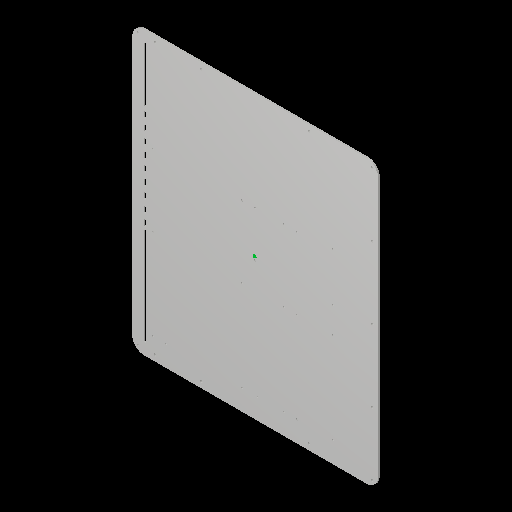
# Autodesk Inventor part: right_panel
Saved by Autodesk Inventor 2022 (Build 260153000, 153)
## iProperties
Created: 2019-10-14
Part Number: right_panel
Material: アルミニウム 6061
Document SubType Name: Modeling
Designer: gisen
Density: 2.7 g/cm^3
Appearance: アルミニウム - フラット
Author: gisen
Autodesk Inventor part; units mm, degrees
ref_plane "YZ Plane" through (0, 0, 0) normal (1, 0, 0) x (0, 1, 0)
ref_plane "XZ Plane" through (0, 0, 0) normal (0, 1, 0) x (-1, 0, 0)
ref_plane "XY Plane" through (0, 0, 0) normal (0, 0, 1) x (1, 0, 0)
sketch "スケッチ1" plane through (0, 0, 0) normal (0, 0, 1) x (1, 0, 0)
  line L0 (-193.5, -245) -> (193.5, -245)
  line L1 (213.5, -225) -> (213.5, 225)
  line L2 (193.5, 245) -> (-193.5, 245)
  line L3 (-213.5, 225) -> (-213.5, -225)
  line L4 (-213.5, -245) -> (213.5, 245) construction
  line L5 (213.5, -245) -> (-213.5, 245) construction
  circle A0 centre (-203.5, 235) radius 2.25
  circle A1 centre (203.5, 235) radius 2.25
  circle A2 centre (-203.5, -235) radius 2.25
  circle A3 centre (203.5, -235) radius 2.25
  arc A4 (-193.5, 245) -> (-213.5, 225) centre (-193.5, 225) ccw
  arc A5 (213.5, 225) -> (193.5, 245) centre (193.5, 225) ccw
  arc A6 (193.5, -245) -> (213.5, -225) centre (193.5, -225) ccw
  arc A7 (-213.5, -225) -> (-193.5, -245) centre (-193.5, -225) ccw
  point P0 (0, 0)
  dimension "d0" = 427
  dimension "d1" = 490
  dimension "d2" = 4.5
  dimension "d3" = 10
  dimension "d4" = 10
  dimension "d5" = 10
  dimension "d6" = 10
  dimension "d7" = 10
  dimension "d8" = 10
  dimension "d9" = 10
  dimension "d10" = 10
  dimension "d11" = 20
  constraints: 12 end point, 8 centre point, 8 point on circle, 8 point on line, 8 tangent, 6 equal radius, 2 midpoint, 2 parallel, 1 horizontal, 1 perpendicular
  measures "d0" distance of L5.end L4.end
  measures "d1" distance of L4.end L5.start
  measures "d2" diameter of A0
  measures "d3" distance from line of A0.centre L2
  measures "d4" distance from line of L3 A0.centre
  measures "d5" distance from line of A1.centre L2
  measures "d6" distance from line of L1 A1.centre
  measures "d7" distance from line of L1 A3.centre
  measures "d8" distance from line of L0 A3.centre
  measures "d9" distance from line of L0 A2.centre
  measures "d10" distance from line of L3 A2.centre
  measures "d11" radius of A4
extrude "押し出し1" add sketch "スケッチ1" along normal blind 3
sketch "スケッチ2" plane through (0, 0, 3) normal (0, 0, 1) x (1, 0, 0)
  circle A0 centre (49.592, 72.9258) radius 1.6
  circle A1 centre (-22.798, 72.9258) radius 1.6
  circle A2 centre (-177.738, 72.9258) radius 1.6
  circle A3 centre (-177.738, -51.5342) radius 1.6
  circle A4 centre (-154.878, -209.0142) radius 1.6
  circle A5 centre (-22.798, -209.0142) radius 1.6
  circle A6 centre (49.592, -209.0142) radius 1.6
  circle A7 centre (49.592, -51.5342) radius 1.6
  circle A8 centre (-22.798, -51.5342) radius 1.6
  circle A9 centre (49.592, -209.0142) radius 2.25 projected
  circle A10 centre (-154.878, -209.0142) radius 2.25 projected
  circle A11 centre (49.592, -51.5342) radius 2.25 projected
  circle A12 centre (49.592, 72.9258) radius 2.25 projected
  circle A13 centre (-22.798, -209.0142) radius 2.25 projected
  circle A14 centre (-22.798, -51.5342) radius 2.25 projected
  circle A15 centre (-22.798, 72.9258) radius 2.25 projected
  circle A16 centre (-177.738, -51.5342) radius 2.25 projected
  circle A17 centre (-177.738, 72.9258) radius 2.25 projected
  point P0 (0, 0)
  dimension "d14" = 3.2
  constraints: 9 centre point, 9 concentric, 8 equal radius
  measures "d14" diameter of A0
extrude "押し出し2" cut sketch "スケッチ2" against normal blind 3 contours A0 | A1 | A2 | A3 | A4 | A5 | A6 | A7 | A8
sketch "スケッチ4" plane through (0, 0, 3) normal (0, 0, 1) x (1, 0, 0)
  line L0 (-193.5, -225) -> (-190.5, -225) projected
  line L1 (-193.5, 225) -> (-193.5, 129.6) projected
  line L2 (-193.5, 129.6) -> (-190.5, 129.6) projected
  line L3 (-190.5, 225) -> (-190.5, 129.6) projected
  line L4 (-193.5, 225) -> (-190.5, 225) projected
  line L5 (-190.5, -40.6067) -> (-189.5, -40.6067)
  line L6 (-189.5, -40.6067) -> (-189.5, -50.8937)
  line L7 (-189.5, -50.8937) -> (-190.5, -50.8937)
  line L8 (-193.5, -225) -> (-193.5, -56.0642) projected
  line L9 (-190.5, -56.0642) -> (-190.5, -225) projected
  line L10 (-190.5, -40.6067) -> (-190.5, -50.8937) construction
  line L11 (-190.5, -50.8937) -> (-193.5, -50.8937)
  line L12 (-193.5, -50.8937) -> (-193.5, -40.6067)
  line L13 (-193.5, -40.6067) -> (-190.5, -40.6067)
  line L14 (-193.5, -56.0642) -> (-190.5, -56.0642) projected
  line L15 (-193.5, -20.2617) -> (-190.5, -20.2617)
  line L16 (-190.5, -20.2617) -> (-189.5, -20.2617)
  line L17 (-189.5, -20.2617) -> (-189.5, -30.5487)
  line L18 (-189.5, -30.5487) -> (-190.5, -30.5487)
  line L19 (-193.5, -30.5487) -> (-193.5, -20.2617)
  line L20 (-190.5, -30.5487) -> (-193.5, -30.5487)
  line L21 (-193.5, 0.0833) -> (-190.5, 0.0833)
  line L22 (-190.5, 0.0833) -> (-189.5, 0.0833)
  line L23 (-189.5, 0.0833) -> (-189.5, -10.2037)
  line L24 (-189.5, -10.2037) -> (-190.5, -10.2037)
  line L25 (-193.5, -10.2037) -> (-193.5, 0.0833)
  line L26 (-190.5, -10.2037) -> (-193.5, -10.2037)
  line L27 (-193.5, 20.4283) -> (-190.5, 20.4283)
  line L28 (-190.5, 20.4283) -> (-189.5, 20.4283)
  line L29 (-189.5, 20.4283) -> (-189.5, 10.1413)
  line L30 (-189.5, 10.1413) -> (-190.5, 10.1413)
  line L31 (-193.5, 10.1413) -> (-193.5, 20.4283)
  line L32 (-190.5, 10.1413) -> (-193.5, 10.1413)
  line L33 (-193.5, 40.7733) -> (-190.5, 40.7733)
  line L34 (-190.5, 40.7733) -> (-189.5, 40.7733)
  line L35 (-189.5, 40.7733) -> (-189.5, 30.4863)
  line L36 (-189.5, 30.4863) -> (-190.5, 30.4863)
  line L37 (-193.5, 30.4863) -> (-193.5, 40.7733)
  line L38 (-190.5, 30.4863) -> (-193.5, 30.4863)
  line L39 (-193.5, 61.1183) -> (-190.5, 61.1183)
  line L40 (-190.5, 61.1183) -> (-189.5, 61.1183)
  line L41 (-189.5, 61.1183) -> (-189.5, 50.8313)
  line L42 (-189.5, 50.8313) -> (-190.5, 50.8313)
  line L43 (-193.5, 50.8313) -> (-193.5, 61.1183)
  line L44 (-190.5, 50.8313) -> (-193.5, 50.8313)
  line L45 (-193.5, 81.4633) -> (-190.5, 81.4633)
  line L46 (-190.5, 81.4633) -> (-189.5, 81.4633)
  line L47 (-189.5, 81.4633) -> (-189.5, 71.1763)
  line L48 (-189.5, 71.1763) -> (-190.5, 71.1763)
  line L49 (-193.5, 71.1763) -> (-193.5, 81.4633)
  line L50 (-190.5, 71.1763) -> (-193.5, 71.1763)
  line L51 (-193.5, 101.8083) -> (-190.5, 101.8083)
  line L52 (-190.5, 101.8083) -> (-189.5, 101.8083)
  line L53 (-189.5, 101.8083) -> (-189.5, 91.5213)
  line L54 (-189.5, 91.5213) -> (-190.5, 91.5213)
  line L55 (-193.5, 91.5213) -> (-193.5, 101.8083)
  line L56 (-190.5, 91.5213) -> (-193.5, 91.5213)
  line L57 (-193.5, 122.1533) -> (-190.5, 122.1533)
  line L58 (-190.5, 122.1533) -> (-189.5, 122.1533)
  line L59 (-189.5, 122.1533) -> (-189.5, 111.8663)
  line L60 (-189.5, 111.8663) -> (-190.5, 111.8663)
  line L61 (-193.5, 111.8663) -> (-193.5, 122.1533)
  line L62 (-190.5, 111.8663) -> (-193.5, 111.8663)
  point P0 (0, 0)
  point P1 (-225, -58.3552)
  point P2 (-222, -58.3552)
  point P3 (-225, -120.4005)
  point P4 (-222, -120.4005)
  dimension "d143" = 20.345
  dimension "d148" = 1
  dimension "d149" = 3
  constraints: 108 end point, 3 perpendicular, 2 collinear, 2 horizontal, 1 vertical, 99 other
  measures "d143" distance of L5.start L15.end
  measures "d148" distance between parallel lines of L10 L6
  measures "d149" distance between parallel lines of L12 L10
extrude "押し出し3" cut sketch "スケッチ4" against normal blind 3
sketch "スケッチ5" plane through (0, 0, 3) normal (0, 0, 1) x (1, 0, 0)
  circle A0 centre (-203.5, 235) radius 2.25 construction
  circle A1 centre (-203.5, -235) radius 2.25 construction
  circle A2 centre (-173.5, -235) radius 2.25
  line L0 (-193.5, -245) -> (193.5, -245) projected
  circle A3 centre (-173.5, 235) radius 2.25
  line L1 (193.5, 245) -> (-193.5, 245) projected
  point P0 (0, 0)
  dimension "d20" = 30
  dimension "d21" = 10
  dimension "d22" = 30
  dimension "d23" = 10
  constraints: 2 centre point, 2 equal radius
  measures "d20" distance of A1.centre A2.centre
  measures "d21" distance from line of L0 A2.centre
  measures "d22" distance of A0.centre A3.centre
  measures "d23" distance from line of L1 A3.centre
extrude "押し出し4" cut sketch "スケッチ5" against normal blind 3
sketch "スケッチ7" plane through (0, 0, 3) normal (0, 0, 1) x (1, 0, 0)
  line L0 (213.5, 225) -> (213.5, -225) projected
  circle A0 centre (-93.5, -235) radius 2.25 projected
  circle A1 centre (203.5, 0) radius 2.25 projected
  circle A2 centre (93.5, -235) radius 2.25 projected
  circle A3 centre (203.5, 125) radius 2.25 projected
  circle A4 centre (-93.5, 235) radius 2.25 projected
  circle A5 centre (-203.5, -125) radius 2.25 projected
  circle A6 centre (-203.5, 0) radius 2.25 projected
  circle A7 centre (93.5, 235) radius 2.25 projected
  circle A8 centre (203.5, -125) radius 2.25 projected
  line L1 (-193.7, 132.4) -> (-190.3, 132.4) projected
  line L2 (-190.3, 132.4) -> (-190.3, 225.2) projected
  line L3 (-190.3, 225.2) -> (-193.7, 225.2) projected
  circle A9 centre (203.5, 235) radius 2.25 projected
  circle A10 centre (-203.5, 235) radius 2.25 projected
  circle A11 centre (203.5, -235) radius 2.25 projected
  circle A12 centre (-203.5, -235) radius 2.25 projected
  line L4 (193.5, -245) -> (-193.5, -245) projected
  arc A13 (-213.5, -225) -> (-193.5, -245) centre (-193.5, -225) ccw projected
  line L5 (-213.5, -225) -> (-213.5, 225) projected
  arc A14 (-193.5, 245) -> (-213.5, 225) centre (-193.5, 225) ccw projected
  line L6 (-193.5, 245) -> (193.5, 245) projected
  arc A15 (213.5, 225) -> (193.5, 245) centre (193.5, 225) ccw projected
  line L7 (213.5, 225) -> (213.5, -225) projected
  arc A16 (193.5, -245) -> (213.5, -225) centre (193.5, -225) ccw projected
  line L8 (-193.7, 225.2) -> (-193.7, 132.4) projected
  circle A17 centre (-203.5, 125) radius 2.25 projected
  point P0 (0, 0)
extrude "押し出し6" cut sketch "スケッチ7" against normal up to surface (3 mm away) contours A0 | A1 | A2 | A3 | A4 | A7 | A8
sketch "スケッチ8" plane through (0, 0, 0) normal (0, 0, -1) x (-1, 0, 0)
  line L0 (-38.275, 130.075) -> (-138.725, 130.075) construction
  line L1 (-138.725, 130.075) -> (-138.725, 199.925) construction
  line L2 (-138.725, 199.925) -> (-38.275, 199.925) construction
  line L3 (-38.275, 199.925) -> (-38.275, 130.075) construction
  line L4 (-38.275, 130.075) -> (-138.725, 199.925) construction
  line L5 (-138.725, 130.075) -> (-38.275, 199.925) construction
  line L6 (193.5, 245) -> (-193.5, 245) construction
  line L7 (-213.5, 225) -> (-213.5, -225) construction
  line L8 (-48.125, 195.86) -> (-124.725, 195.86) construction
  line L9 (-124.725, 195.86) -> (-124.725, 134.14) construction
  line L10 (-124.725, 134.14) -> (-48.125, 134.14) construction
  line L11 (-48.125, 134.14) -> (-48.125, 195.86) construction
  line L12 (-48.125, 195.86) -> (-124.725, 134.14) construction
  line L13 (-124.725, 195.86) -> (-48.125, 134.14) construction
  line L14 (-86.425, 165) -> (-88.5, 165) construction
  circle A0 centre (-48.125, 134.14) radius 1.6
  circle A1 centre (-48.125, 195.86) radius 1.6
  circle A2 centre (-124.725, 195.86) radius 1.6
  circle A3 centre (-124.725, 134.14) radius 1.6
  point P0 (0, 0)
  dimension "d40" = 69.85
  dimension "d41" = 100.45
  dimension "d42" = 80
  dimension "d43" = 125
  dimension "d44" = 61.72
  dimension "d45" = 90.6
  dimension "d46" = 14
  dimension "d47" = 3.2
  dimension "d48" = 3.2
  dimension "d49" = 3.2
  dimension "d50" = 3.2
  constraints: 26 end point, 4 centre point, 4 coincident, 4 midpoint, 4 parallel, 3 horizontal, 2 perpendicular
  measures "d40" distance of L0.end L1.end
  measures "d41" distance of L0.start L0.end
  measures "d42" distance from line of L6 L14.end
  measures "d43" distance from line of L7 L14.end
  measures "d44" distance of L10.end L8.start
  measures "d45" distance between parallel lines of L1 L11
  measures "d46" distance between parallel lines of L1 L9
  measures "d47" diameter of A0
  measures "d48" diameter of A1
  measures "d49" diameter of A2
  measures "d50" diameter of A3
extrude "押し出し7" [suppressed]
sketch "スケッチ9" plane through (0, 0, 0) normal (0, 0, -1) x (-1, 0, 0)
  circle A0 centre (154.878, -209.0142) radius 1.6 construction
  circle A1 centre (22.798, -209.0142) radius 1.6 construction
  circle A2 centre (-49.592, -209.0142) radius 1.6 construction
  circle A3 centre (177.738, -51.5342) radius 1.6 construction
  circle A4 centre (177.738, 72.9258) radius 1.6 construction
  circle A5 centre (22.798, 72.9258) radius 1.6 construction
  circle A6 centre (-49.592, 72.9258) radius 1.6 construction
  circle A7 centre (22.798, -51.5342) radius 1.6 construction
  circle A8 centre (-49.592, -51.5342) radius 1.6 construction
  line L0 (187.898, -215.3642) -> (-83.882, -215.3642) construction
  line L1 (-83.882, -215.3642) -> (-83.882, 89.4358) construction
  line L2 (-83.882, 89.4358) -> (187.898, 89.4358) construction
  line L3 (187.898, 89.4358) -> (187.898, -215.3642) construction
  point P0 (0, 0)
  dimension "d53" = 6.35
  dimension "d54" = 33.02
  dimension "d55" = 304.8
  dimension "d56" = 271.78
  constraints: 8 end point, 2 parallel, 1 horizontal, 1 perpendicular
  measures "d53" distance from line of A0.centre L0
  measures "d54" distance from line of L3 A0.centre
  measures "d55" distance of L2.end L0.start
  measures "d56" distance of L0.start L0.end
sketch "スケッチ10" plane through (0, 0, 0) normal (0, 0, -1) x (-1, 0, 0)
  line L0 (187.898, -215.3642) -> (-142.302, -215.3642) construction
  line L1 (-142.302, -215.3642) -> (-142.302, 89.4358) construction
  line L2 (-142.302, 89.4358) -> (187.898, 89.4358) construction
  line L3 (187.898, 89.4358) -> (187.898, -215.3642) construction
  circle A0 centre (177.738, 72.9258) radius 1.6 construction
  circle A1 centre (-203.5, -125) radius 2.25 projected
  circle A2 centre (-134.682, 78.0058) radius 1.6
  circle A3 centre (177.738, 72.9258) radius 1.6 construction
  line L4 (177.738, 72.9258) -> (22.798, 72.9258) construction
  circle A4 centre (22.798, 72.9258) radius 1.6 construction
  circle A5 centre (22.798, 72.9258) radius 1.6 construction
  line L5 (22.798, 72.9258) -> (-49.592, 72.9258) construction
  line L6 (-49.592, 72.9258) -> (-72.452, 72.9258) construction
  circle A6 centre (-49.592, 72.9258) radius 1.6
  circle A7 centre (-72.452, 72.9258) radius 1.6
  line L7 (-134.682, 78.0058) -> (-134.682, -5.8142) construction
  line L8 (-134.682, -5.8142) -> (-134.682, -51.5342) construction
  line L9 (-134.682, -51.5342) -> (-134.682, -208.9142) construction
  circle A8 centre (-134.682, -5.8142) radius 1.6
  circle A9 centre (-134.682, -51.5342) radius 1.6
  circle A10 centre (-134.682, -208.9142) radius 1.6
  line L10 (-134.682, -5.8142) -> (-0.062, -5.8142) construction
  circle A11 centre (-0.062, -5.8142) radius 1.6
  line L11 (-0.062, -5.8142) -> (-0.062, 72.9258) construction
  circle A12 centre (-0.062, 72.9258) radius 1.6
  line L12 (177.738, 72.9258) -> (177.738, -209.0142) construction
  circle A13 centre (154.878, -209.0142) radius 1.6 construction
  line L13 (177.738, -209.0142) -> (154.878, -209.0142) construction
  circle A14 centre (177.738, -209.0142) radius 1.6
  line L14 (-72.452, 72.9258) -> (-72.452, -209.0142) construction
  line L15 (-72.452, -209.0142) -> (-49.592, -209.0142) construction
  circle A15 centre (-49.592, -51.5342) radius 1.6 construction
  line L16 (-49.592, -51.5342) -> (-72.452, -51.5342) construction
  circle A16 centre (-49.592, -209.0142) radius 1.6 construction
  circle A17 centre (-72.452, -51.5342) radius 1.6
  circle A18 centre (-72.452, -209.0142) radius 1.6
  line L17 (-49.592, -209.0142) -> (154.878, -209.0142) construction
  circle A19 centre (-3.872, -209.0142) radius 1.6
  point P0 (0, 0)
  dimension "d57" = 330.2
  dimension "d58" = 304.8
  dimension "d59" = 10.16
  dimension "d60" = 16.51
  dimension "d61" = 61.198
  dimension "d62" = 5.08
  dimension "d63" = 312.42
  dimension "d64" = 154.94
  dimension "d65" = 227.33
  dimension "d66" = 250.19
  dimension "d67" = 78.74
  dimension "d68" = 124.46
  dimension "d69" = 281.84
  dimension "d70" = 177.8
  dimension "d71" = 134.62
  dimension "d72" = 16.51
  dimension "d73" = 181.61
  dimension "d74" = 3.2
  constraints: 36 end point, 14 centre point, 13 coincident, 13 equal radius, 6 point on line, 5 horizontal, 4 perpendicular, 4 vertical, 2 parallel
  measures "d57" distance of L0.start L0.end
  measures "d58" distance of L0.end L1.end
  measures "d59" distance from line of A0.centre L3
  measures "d60" distance from line of L2 A0.centre
  measures "d61" distance from line of L1 A1.centre
  measures "d62" vertical distance of A0.centre L7.start
  measures "d63" horizontal distance of A0.centre L7.start
  measures "d64" distance of L4.start L4.end
  measures "d65" distance of L5.end L4.start
  measures "d66" distance of L4.start L6.end
  measures "d67" vertical distance of L10.start A0.centre
  measures "d68" vertical distance of L8.end A0.centre
  measures "d69" vertical distance of L4.start L9.end
  measures "d70" horizontal distance of L4.start L10.end
  measures "d71" distance of L10.start L10.end
  measures "d72" distance from line of L2 L11.end
  measures "d73" distance from line of L12 A19.centre
  measures "d74" diameter of A0
extrude "押し出し8" cut sketch "スケッチ10" against normal blind 10 contours A2 | A7 | A8 | A9 | A10 | A11 | A12 | A14 | A17 | A18 | A19
sketch "スケッチ11" plane through (0, 0, 3) normal (0, 0, 1) x (1, 0, 0)
  point P0 (0, 0)
sketch "スケッチ12" plane through (0, 0, 0) normal (0, 0, -1) x (-1, 0, 0)
  line L0 (190.5, 225) -> (193.5, 225) construction
  line L1 (190.5, 129.6) -> (190.5, 225) construction
  line L2 (193.5, 225) -> (193.5, 129.6) construction
  line L3 (193.5, 129.6) -> (190.5, 129.6) construction
  line L4 (189.5, -40.6067) -> (193.5, -40.6067) construction
  line L5 (189.5, -50.8937) -> (189.5, -40.6067) construction
  line L6 (193.5, -50.8937) -> (189.5, -50.8937) construction
  line L7 (193.5, -40.6067) -> (193.5, -50.8937) construction
  line L8 (190.5, -56.0642) -> (193.5, -56.0642) construction
  line L9 (190.5, -225) -> (190.5, -56.0642) construction
  line L10 (193.5, -56.0642) -> (193.5, -225) construction
  line L11 (193.5, -225) -> (190.5, -225) construction
  line L12 (190.3, -225.2) -> (190.3, -55.8642)
  line L13 (190.3, -55.8642) -> (193.7, -55.8642)
  line L14 (193.7, -55.8642) -> (193.7, -225.2)
  line L15 (193.7, -225.2) -> (190.3, -225.2)
  line L16 (193.7, -51.0937) -> (189.3, -51.0937)
  line L17 (189.3, -51.0937) -> (189.3, -40.4067)
  line L18 (189.3, -40.4067) -> (193.7, -40.4067)
  line L19 (193.7, -40.4067) -> (193.7, -51.0937)
  line L20 (190.3, 129.4) -> (190.3, 225.2)
  line L21 (190.3, 225.2) -> (193.7, 225.2)
  line L22 (193.7, 225.2) -> (193.7, 129.4)
  line L23 (193.7, 129.4) -> (190.3, 129.4)
  line L24 (193.7, -30.7487) -> (189.3, -30.7487)
  line L25 (193.7, -20.0617) -> (193.7, -30.7487)
  line L26 (189.3, -20.0617) -> (193.7, -20.0617)
  line L27 (189.3, -30.7487) -> (189.3, -20.0617)
  line L28 (193.7, -10.4037) -> (189.3, -10.4037)
  line L29 (193.7, 0.2833) -> (193.7, -10.4037)
  line L30 (189.3, 0.2833) -> (193.7, 0.2833)
  line L31 (189.3, -10.4037) -> (189.3, 0.2833)
  line L32 (193.7, 9.9413) -> (189.3, 9.9413)
  line L33 (193.7, 20.6283) -> (193.7, 9.9413)
  line L34 (189.3, 20.6283) -> (193.7, 20.6283)
  line L35 (189.3, 9.9413) -> (189.3, 20.6283)
  line L36 (193.7, 30.2863) -> (189.3, 30.2863)
  line L37 (193.7, 40.9733) -> (193.7, 30.2863)
  line L38 (189.3, 40.9733) -> (193.7, 40.9733)
  line L39 (189.3, 30.2863) -> (189.3, 40.9733)
  line L40 (193.7, 50.6313) -> (189.3, 50.6313)
  line L41 (193.7, 61.3183) -> (193.7, 50.6313)
  line L42 (189.3, 61.3183) -> (193.7, 61.3183)
  line L43 (189.3, 50.6313) -> (189.3, 61.3183)
  line L44 (193.7, 70.9763) -> (189.3, 70.9763)
  line L45 (193.7, 81.6633) -> (193.7, 70.9763)
  line L46 (189.3, 81.6633) -> (193.7, 81.6633)
  line L47 (189.3, 70.9763) -> (189.3, 81.6633)
  line L48 (193.7, 91.3213) -> (189.3, 91.3213)
  line L49 (193.7, 102.0083) -> (193.7, 91.3213)
  line L50 (189.3, 102.0083) -> (193.7, 102.0083)
  line L51 (189.3, 91.3213) -> (189.3, 102.0083)
  line L52 (193.7, 111.6663) -> (189.3, 111.6663)
  line L53 (193.7, 122.3533) -> (193.7, 111.6663)
  line L54 (189.3, 122.3533) -> (193.7, 122.3533)
  line L55 (189.3, 111.6663) -> (189.3, 122.3533)
  point P0 (0, 0)
  point P1 (176.138, -51.5342)
  point P2 (176.138, -51.5342)
  dimension "d128" = 0.2
  dimension "d129" = 0.2
  dimension "d138" = 0.2
  dimension "d152" = 20.345
  constraints: 88 end point, 1 collinear, 1 perpendicular, 1 vertical, 73 other
  measures "d128" distance between parallel lines of L11 L15
  measures "d138" distance between parallel lines of L3 L23
  measures "d152" distance of L16.start L24.start
extrude "押し出し9" cut sketch "スケッチ12" against normal through all
equation "\"d5\" = d3"
equation "\"d6\" = d4"
equation "\"d7\" = d6"
equation "\"d8\" = d5"
equation "\"d9\" = d8"
equation "\"d10\" = d7"
